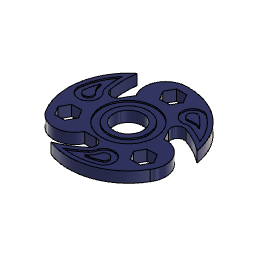
Fidget Spinner (Autodesk Fusion 360 design; units mm, degrees)
Autodesk Fusion 360 part; units mm, degrees
sketch "Sketch1" plane through (0, 0, 0) normal (0, 0, 1) x (1, 0, 0)
  circle A0 centre (0, 0) radius 4
  circle A1 centre (0, 0) radius 11
  circle A2 centre (0, 0) radius 13.5
  circle A3 centre (0, 0) radius 17.5
  line L0 (-18.6674, 12.667) -> (-14.3305, 20.1788)
  line L1 (20.3037, 9.833) -> (24.5374, 2.5)
  line L2 (-10.1036, -22.5) -> (-1.6363, -22.5)
  arc A4 (38.9711, 22.5) -> (0, 45) centre (0, 0) ccw
  arc A5 (44.4373, 7.0943) -> (38.9711, 22.5) centre (0, 0) ccw
  arc A6 (0, 45) -> (-14.3305, 20.1788) centre (-0.9803, 29.0185) ccw
  arc A7 (44.4373, 7.0943) -> (26.3003, 17.0471) centre (4.9389, -43.3819) ccw
  line L3 (-3.4682, 39.5482) -> (-7.0418, 32.948)
  line L4 (-7.0418, 32.948) -> (-3.1126, 26.5531)
  line L5 (-3.1126, 26.5531) -> (4.3902, 26.7584)
  line L6 (4.3902, 26.7584) -> (7.9637, 33.3586)
  line L7 (7.9637, 33.3586) -> (4.0345, 39.7535)
  line L8 (4.0345, 39.7535) -> (-3.4682, 39.5482)
  arc A8 (26.3003, 17.0471) -> (20.3037, 9.833) centre (24.6338, 12.333) ccw
  arc A9 (-38.9711, -22.5) -> (-10.3101, -22.5) centre (-24.6406, -15.3583) ccw
  arc A10 (-38.9711, 22.5) -> (-38.9711, -22.5) centre (0, 0) ccw
  line L9 (-32.8713, -9.7825) -> (-36.4448, -16.3828)
  line L10 (-36.4448, -16.3828) -> (-32.5156, -22.7777)
  line L11 (-32.5156, -22.7777) -> (-25.0129, -22.5723)
  line L12 (-25.0129, -22.5723) -> (-21.4394, -15.9721)
  line L13 (-21.4394, -15.9721) -> (-25.3686, -9.5772)
  line L14 (-25.3686, -9.5772) -> (-32.8713, -9.7825)
  arc A11 (-28.3625, 34.9366) -> (-38.9711, 22.5) centre (0, 0) ccw
  arc A12 (-28.3625, 34.9366) -> (-27.9133, 14.2531) centre (35.1004, 25.9682) ccw
  arc A13 (-27.9133, 14.2531) -> (-18.6674, 12.667) centre (-22.9976, 15.167) ccw
  line L15 (-18.6674, 12.667) -> (-14.4338, 20)
  line L16 (24.5374, 2.5) -> (20.3037, 9.833)
  line L17 (-1.6363, -22.5) -> (-10.3101, -22.5)
  arc A14 (38.9711, -22.5) -> (24.6406, 2.3212) centre (25.6209, -13.6603) ccw
  arc A15 (0, -45) -> (38.9711, -22.5) centre (0, 0) ccw
  line L18 (24.9076, -23.5761) -> (32.4103, -23.3708)
  line L19 (32.4103, -23.3708) -> (35.9839, -16.7705)
  line L20 (35.9839, -16.7705) -> (32.0547, -10.3756)
  line L21 (32.0547, -10.3756) -> (24.5519, -10.581)
  line L22 (24.5519, -10.581) -> (20.9784, -17.1812)
  line L23 (20.9784, -17.1812) -> (24.9076, -23.5761)
  arc A16 (-16.0748, -42.031) -> (0, -45) centre (0, 0) ccw
  arc A17 (-16.0748, -42.031) -> (1.6131, -31.3002) centre (-40.0393, 17.4137) ccw
  arc A18 (1.6131, -31.3002) -> (-1.6363, -22.5) centre (-1.6363, -27.5) ccw
  line L24 (-1.6363, -22.5) -> (-10.1036, -22.5)
  line L25 (-14.4338, 20) -> (-18.6674, 12.667)
  line L26 (20.3037, 9.833) -> (24.6406, 2.3212)
  dimension "d2" = 8
  dimension "d4" = 22
  dimension "d5" = 2.5
  dimension "d6" = 35
  dimension "d12" = 22
  dimension "d13" = 8
  dimension "d14" = 5
  constraint coincident A0.centre A1.centre
  constraint coincident A6.start A4
  constraint tangent L1 A8
  constraint tangent A7 A8
  measures "d2" diameter of A0
  measures "d4" diameter of A1
  measures "d6" diameter of A3
  measures "d12" diameter of A1
  measures "d13" diameter of A0
  measures "d14" radius of A8
sketch "Sketch2" plane through (0, 0, 0) normal (0, 0, 1) x (1, 0, 0)
extrude "Extrude1" add sketch "Sketch1" along normal blind 8 contours A2 | A3 | L0 L1 L2 A4 A5 A6 A7 A8 A9 A10 A11 A12 A13 L15 L16 L17 A14 A15 A16 A17 A18 L24 L25 L26
sketch "Sketch3" plane through (0, 0, 8) normal (0, 0, 1) x (-1, 0, 0)
  line L0 (32.8713, 9.7825) -> (25.3686, 9.5772)
  line L1 (25.3686, 9.5772) -> (21.4394, 15.9721)
  line L2 (21.4394, 15.9721) -> (25.0129, 22.5723)
  line L3 (25.0129, 22.5723) -> (32.5156, 22.7777)
  line L4 (32.5156, 22.7777) -> (36.4448, 16.3828)
  line L5 (36.4448, 16.3828) -> (32.8713, 9.7825)
  line L6 (3.4682, -39.5482) -> (-4.0345, -39.7535)
  line L7 (-4.0345, -39.7535) -> (-7.9637, -33.3586)
  line L8 (-7.9637, -33.3586) -> (-4.3902, -26.7584)
  line L9 (-4.3902, -26.7584) -> (3.1126, -26.5531)
  line L10 (3.1126, -26.5531) -> (7.0418, -32.948)
  line L11 (7.0418, -32.948) -> (3.4682, -39.5482)
  circle A0 centre (0, 0) radius 11
  line L12 (-24.9076, 23.5761) -> (-20.9784, 17.1812)
  line L13 (-20.9784, 17.1812) -> (-24.5519, 10.581)
  line L14 (-24.5519, 10.581) -> (-32.0547, 10.3756)
  line L15 (-32.0547, 10.3756) -> (-35.9839, 16.7705)
  line L16 (-35.9839, 16.7705) -> (-32.4103, 23.3708)
  line L17 (-32.4103, 23.3708) -> (-24.9076, 23.5761)
  arc A1 (-44.4373, -7.0943) -> (0, -45) centre (0, 0) ccw
  arc A2 (0, -45) -> (14.3305, -20.1788) centre (0.9803, -29.0185) ccw
  line L18 (14.3305, -20.1788) -> (18.6674, -12.667)
  arc A3 (27.9133, -14.2531) -> (18.6674, -12.667) centre (22.9976, -15.167) ccw
  arc A4 (28.3625, -34.9366) -> (27.9133, -14.2531) centre (-35.1004, -25.9682) ccw
  arc A5 (28.3625, -34.9366) -> (38.9711, 22.5) centre (0, 0) ccw
  arc A6 (38.9711, 22.5) -> (10.3101, 22.5) centre (24.6406, 15.3583) ccw
  line L19 (10.3101, 22.5) -> (1.6363, 22.5)
  arc A7 (-1.6131, 31.3002) -> (1.6363, 22.5) centre (1.6363, 27.5) ccw
  arc A8 (16.0748, 42.031) -> (-1.6131, 31.3002) centre (40.0393, -17.4137) ccw
  arc A9 (16.0748, 42.031) -> (-38.9711, 22.5) centre (0, 0) ccw
  arc A10 (-38.9711, 22.5) -> (-24.6406, -2.3212) centre (-25.6209, 13.6603) ccw
  line L20 (-24.6406, -2.3212) -> (-20.3037, -9.833)
  arc A11 (-26.3003, -17.0471) -> (-20.3037, -9.833) centre (-24.6338, -12.333) ccw
  arc A12 (-44.4373, -7.0943) -> (-26.3003, -17.0471) centre (-4.9389, 43.3819) ccw
  arc A13 (30.8628, -13.7048) -> (28.0927, -8.9994) centre (22.9976, -15.167) ccw
  arc A14 (31.9813, -27.2249) -> (30.8628, -13.7048) centre (-35.1004, -25.9682) ccw
  arc A15 (31.9813, -27.2249) -> (41.8312, -3.7617) centre (0, 0) ccw
  arc A16 (7.5868, 41.3091) -> (-3.5627, 33.5804) centre (40.0393, -17.4137) ccw
  arc A17 (41.8312, -3.7617) -> (29.2995, -10.239) centre (34.1663, -4.2937) ccw
  arc A18 (31.9813, -27.2249) -> (41.8312, -3.7617) centre (0, 0) ccw
  arc A19 (7.5868, 41.3091) -> (-17.6578, 38.1078) centre (0, 0) ccw
  arc A20 (7.5868, 41.3091) -> (-3.5627, 33.5804) centre (40.0393, -17.4137) ccw
  arc A21 (-17.6578, 38.1078) -> (-5.7825, 30.4936) centre (-13.3647, 31.7358) ccw
  arc A22 (-3.5627, 33.5804) -> (-6.2526, 28.8287) centre (1.6363, 27.5) ccw
  arc A23 (-39.5681, -14.0842) -> (-24.1734, -34.346) centre (0, 0) ccw
  arc A24 (-39.5681, -14.0842) -> (-27.3001, -19.8756) centre (-4.9389, 43.3819) ccw
  arc A25 (-24.1734, -34.346) -> (-23.517, -20.2546) centre (-20.8016, -27.4421) ccw
  arc A26 (-27.3001, -19.8756) -> (-21.8401, -19.8293) centre (-24.6338, -12.333) ccw
  dimension "d22" = 360
  constraint coincident A13 A17.end
  constraint concentric A3 A13
  constraint concentric A4 A14
  constraint concentric A5 A15
  constraint concentric A8 A16
  constraint tangent A13 A14
  constraint coincident A17 A13.end
extrude "Extrude2" cut sketch "Sketch3" against normal blind 1 contours A13 A14 A15 A17 A18 | A16 A19 A20 A21 A22 | A23 A24 A25 A26
sketch "Sketch4" plane through (0, 0, 8) normal (0, 0, 1) x (-1, 0, 0)
  arc A0 (31.9813, -27.2249) -> (41.8312, -3.7617) centre (0, 0) ccw
  arc A1 (31.9813, -27.2249) -> (30.8628, -13.7048) centre (-35.1004, -25.9682) ccw
  arc A2 (30.8628, -13.7048) -> (28.0927, -8.9994) centre (22.9976, -15.167) ccw
  arc A3 (41.8312, -3.7617) -> (28.0927, -8.9994) centre (34.1663, -4.2937) ccw
  arc A4 (-24.1734, -34.346) -> (-21.8401, -19.8293) centre (-20.8016, -27.4421) ccw
  arc A5 (-39.5681, -14.0842) -> (-24.1734, -34.346) centre (0, 0) ccw
  arc A6 (-39.5681, -14.0842) -> (-27.3001, -19.8756) centre (-4.9389, 43.3819) ccw
  arc A7 (-27.3001, -19.8756) -> (-21.8401, -19.8293) centre (-24.6338, -12.333) ccw
  arc A8 (-17.6578, 38.1078) -> (-6.2526, 28.8287) centre (-13.3647, 31.7358) ccw
  arc A9 (7.5868, 41.3091) -> (-17.6578, 38.1078) centre (0, 0) ccw
  arc A10 (7.5868, 41.3091) -> (-3.5627, 33.5804) centre (40.0393, -17.4137) ccw
  arc A11 (-3.5627, 33.5804) -> (-6.2526, 28.8287) centre (1.6363, 27.5) ccw
  line L0 (32.8713, 9.7825) -> (25.3686, 9.5772)
  line L1 (25.3686, 9.5772) -> (21.4394, 15.9721)
  line L2 (21.4394, 15.9721) -> (25.0129, 22.5723)
  line L3 (25.0129, 22.5723) -> (32.5156, 22.7777)
  line L4 (32.5156, 22.7777) -> (36.4448, 16.3828)
  line L5 (36.4448, 16.3828) -> (32.8713, 9.7825)
  line L6 (3.4682, -39.5482) -> (-4.0345, -39.7535)
  line L7 (-4.0345, -39.7535) -> (-7.9637, -33.3586)
  line L8 (-7.9637, -33.3586) -> (-4.3902, -26.7584)
  line L9 (-4.3902, -26.7584) -> (3.1126, -26.5531)
  line L10 (3.1126, -26.5531) -> (7.0418, -32.948)
  line L11 (7.0418, -32.948) -> (3.4682, -39.5482)
  circle A12 centre (0, 0) radius 11
  line L12 (-24.9076, 23.5761) -> (-20.9784, 17.1812)
  line L13 (-20.9784, 17.1812) -> (-24.5519, 10.581)
  line L14 (-24.5519, 10.581) -> (-32.0547, 10.3756)
  line L15 (-32.0547, 10.3756) -> (-35.9839, 16.7705)
  line L16 (-35.9839, 16.7705) -> (-32.4103, 23.3708)
  line L17 (-32.4103, 23.3708) -> (-24.9076, 23.5761)
  arc A13 (-44.4373, -7.0943) -> (0, -45) centre (0, 0) ccw
  arc A14 (0, -45) -> (14.3305, -20.1788) centre (0.9803, -29.0185) ccw
  line L18 (14.3305, -20.1788) -> (18.6674, -12.667)
  arc A15 (27.9133, -14.2531) -> (18.6674, -12.667) centre (22.9976, -15.167) ccw
  arc A16 (28.3625, -34.9366) -> (27.9133, -14.2531) centre (-35.1004, -25.9682) ccw
  arc A17 (28.3625, -34.9366) -> (38.9711, 22.5) centre (0, 0) ccw
  arc A18 (38.9711, 22.5) -> (10.3101, 22.5) centre (24.6406, 15.3583) ccw
  line L19 (10.3101, 22.5) -> (1.6363, 22.5)
  arc A19 (-1.6131, 31.3002) -> (1.6363, 22.5) centre (1.6363, 27.5) ccw
  arc A20 (16.0748, 42.031) -> (-1.6131, 31.3002) centre (40.0393, -17.4137) ccw
  arc A21 (16.0748, 42.031) -> (-38.9711, 22.5) centre (0, 0) ccw
  arc A22 (-38.9711, 22.5) -> (-24.6406, -2.3212) centre (-25.6209, 13.6603) ccw
  line L20 (-24.6406, -2.3212) -> (-20.3037, -9.833)
  arc A23 (-26.3003, -17.0471) -> (-20.3037, -9.833) centre (-24.6338, -12.333) ccw
  arc A24 (-44.4373, -7.0943) -> (-26.3003, -17.0471) centre (-4.9389, 43.3819) ccw
  circle A25 centre (0, 0) radius 15
  circle A26 centre (0, 0) radius 20
  constraint coincident A0.centre A5.centre
  constraint concentric A25 A26
sketch "Sketch5" plane through (0, 0, 8) normal (0, 0, 1) x (-1, 0, 0)
extrude "Extrude3" cut sketch "Sketch4" against normal blind 1 contours A26
sketch "Sketch6" plane through (0, 0, 0) normal (0, 0, -1) x (1, 0, 0)
  line L0 (-25.3686, 9.5772) -> (-32.8713, 9.7825)
  line L1 (-32.8713, 9.7825) -> (-36.4448, 16.3828)
  line L2 (-36.4448, 16.3828) -> (-32.5156, 22.7777)
  line L3 (-32.5156, 22.7777) -> (-25.0129, 22.5723)
  line L4 (-25.0129, 22.5723) -> (-21.4394, 15.9721)
  line L5 (-21.4394, 15.9721) -> (-25.3686, 9.5772)
  line L6 (4.0345, -39.7535) -> (-3.4682, -39.5482)
  line L7 (-3.4682, -39.5482) -> (-7.0418, -32.948)
  line L8 (-7.0418, -32.948) -> (-3.1126, -26.5531)
  line L9 (-3.1126, -26.5531) -> (4.3902, -26.7584)
  line L10 (4.3902, -26.7584) -> (7.9637, -33.3586)
  line L11 (7.9637, -33.3586) -> (4.0345, -39.7535)
  circle A0 centre (0, 0) radius 11
  line L12 (20.9784, 17.1812) -> (24.9076, 23.5761)
  line L13 (24.9076, 23.5761) -> (32.4103, 23.3708)
  line L14 (32.4103, 23.3708) -> (35.9839, 16.7705)
  line L15 (35.9839, 16.7705) -> (32.0547, 10.3756)
  line L16 (32.0547, 10.3756) -> (24.5519, 10.581)
  line L17 (24.5519, 10.581) -> (20.9784, 17.1812)
  arc A1 (0, -45) -> (44.4373, -7.0943) centre (0, 0) ccw
  arc A2 (26.3003, -17.0471) -> (44.4373, -7.0943) centre (4.9389, 43.3819) ccw
  arc A3 (20.3037, -9.833) -> (26.3003, -17.0471) centre (24.6338, -12.333) ccw
  line L18 (20.3037, -9.833) -> (24.6406, -2.3212)
  arc A4 (24.6406, -2.3212) -> (38.9711, 22.5) centre (25.6209, 13.6603) ccw
  arc A5 (38.9711, 22.5) -> (-16.0748, 42.031) centre (0, 0) ccw
  arc A6 (1.6131, 31.3002) -> (-16.0748, 42.031) centre (-40.0393, -17.4137) ccw
  arc A7 (-1.6363, 22.5) -> (1.6131, 31.3002) centre (-1.6363, 27.5) ccw
  line L19 (-1.6363, 22.5) -> (-10.3101, 22.5)
  arc A8 (-10.3101, 22.5) -> (-38.9711, 22.5) centre (-24.6406, 15.3583) ccw
  arc A9 (-38.9711, 22.5) -> (-28.3625, -34.9366) centre (0, 0) ccw
  arc A10 (-27.9133, -14.2531) -> (-28.3625, -34.9366) centre (35.1004, -25.9682) ccw
  arc A11 (-18.6674, -12.667) -> (-27.9133, -14.2531) centre (-22.9976, -15.167) ccw
  line L20 (-18.6674, -12.667) -> (-14.3305, -20.1788)
  arc A12 (-14.3305, -20.1788) -> (0, -45) centre (-0.9803, -29.0185) ccw
  arc A13 (-28.2531, -9.1355) -> (-30.8628, -13.7048) centre (-22.9976, -15.167) ccw
  arc A14 (-30.8628, -13.7048) -> (-31.9813, -27.2249) centre (35.1004, -25.9682) ccw
  arc A15 (-41.8312, -3.7617) -> (-31.9813, -27.2249) centre (0, 0) ccw
  arc A16 (-29.2995, -10.239) -> (-41.8312, -3.7617) centre (-34.2643, -4.4832) ccw
  arc A17 (22.0381, -19.9001) -> (27.3001, -19.8756) centre (24.6338, -12.333) ccw
  arc A18 (27.3001, -19.8756) -> (39.5681, -14.0842) centre (4.9389, 43.3819) ccw
  arc A19 (24.1734, -34.346) -> (39.5681, -14.0842) centre (0, 0) ccw
  arc A20 (23.517, -20.2546) -> (24.1734, -34.346) centre (21.0147, -27.4321) ccw
  arc A21 (6.215, 29.0357) -> (3.5627, 33.5804) centre (-1.6363, 27.5) ccw
  arc A22 (3.5627, 33.5804) -> (-7.5868, 41.3091) centre (-40.0393, -17.4137) ccw
  arc A23 (17.6578, 38.1078) -> (-7.5868, 41.3091) centre (0, 0) ccw
  arc A24 (5.7825, 30.4936) -> (17.6578, 38.1078) centre (13.2496, 31.9154) ccw
  dimension "d29" = 360
  constraint coincident A13 A16.start
  constraint concentric A11 A13
  constraint concentric A10 A14
  constraint concentric A9 A15
  constraint tangent A13 A14
  constraint coincident A16 A13.start
extrude "Extrude4" cut sketch "Sketch6" against normal blind 1 contours A13 A14 A15 A16 | A17 A18 A19 A20 | A21 A22 A23 A24
sketch "Sketch7" plane through (0, 0, 0) normal (0, 0, -1) x (1, 0, 0)
  arc A0 (3.5627, 33.5804) -> (-7.5868, 41.3091) centre (-40.0393, -17.4137) ccw
  arc A1 (17.6578, 38.1078) -> (-7.5868, 41.3091) centre (0, 0) ccw
  arc A2 (6.215, 29.0357) -> (17.6578, 38.1078) centre (13.2496, 31.9154) ccw
  arc A3 (6.215, 29.0357) -> (3.5627, 33.5804) centre (-1.6363, 27.5) ccw
  arc A4 (27.3001, -19.8756) -> (39.5681, -14.0842) centre (4.9389, 43.3819) ccw
  arc A5 (24.1734, -34.346) -> (39.5681, -14.0842) centre (0, 0) ccw
  arc A6 (22.0381, -19.9001) -> (24.1734, -34.346) centre (21.0147, -27.4321) ccw
  arc A7 (22.0381, -19.9001) -> (27.3001, -19.8756) centre (24.6338, -12.333) ccw
  arc A8 (-30.8628, -13.7048) -> (-31.9813, -27.2249) centre (35.1004, -25.9682) ccw
  arc A9 (-41.8312, -3.7617) -> (-31.9813, -27.2249) centre (0, 0) ccw
  arc A10 (-28.2531, -9.1355) -> (-41.8312, -3.7617) centre (-34.2643, -4.4832) ccw
  arc A11 (-28.2531, -9.1355) -> (-30.8628, -13.7048) centre (-22.9976, -15.167) ccw
  line L0 (-25.3686, 9.5772) -> (-32.8713, 9.7825)
  line L1 (-32.8713, 9.7825) -> (-36.4448, 16.3828)
  line L2 (-36.4448, 16.3828) -> (-32.5156, 22.7777)
  line L3 (-32.5156, 22.7777) -> (-25.0129, 22.5723)
  line L4 (-25.0129, 22.5723) -> (-21.4394, 15.9721)
  line L5 (-21.4394, 15.9721) -> (-25.3686, 9.5772)
  line L6 (4.0345, -39.7535) -> (-3.4682, -39.5482)
  line L7 (-3.4682, -39.5482) -> (-7.0418, -32.948)
  line L8 (-7.0418, -32.948) -> (-3.1126, -26.5531)
  line L9 (-3.1126, -26.5531) -> (4.3902, -26.7584)
  line L10 (4.3902, -26.7584) -> (7.9637, -33.3586)
  line L11 (7.9637, -33.3586) -> (4.0345, -39.7535)
  circle A12 centre (0, 0) radius 11
  line L12 (20.9784, 17.1812) -> (24.9076, 23.5761)
  line L13 (24.9076, 23.5761) -> (32.4103, 23.3708)
  line L14 (32.4103, 23.3708) -> (35.9839, 16.7705)
  line L15 (35.9839, 16.7705) -> (32.0547, 10.3756)
  line L16 (32.0547, 10.3756) -> (24.5519, 10.581)
  line L17 (24.5519, 10.581) -> (20.9784, 17.1812)
  arc A13 (0, -45) -> (44.4373, -7.0943) centre (0, 0) ccw
  arc A14 (26.3003, -17.0471) -> (44.4373, -7.0943) centre (4.9389, 43.3819) ccw
  arc A15 (20.3037, -9.833) -> (26.3003, -17.0471) centre (24.6338, -12.333) ccw
  line L18 (20.3037, -9.833) -> (24.6406, -2.3212)
  arc A16 (24.6406, -2.3212) -> (38.9711, 22.5) centre (25.6209, 13.6603) ccw
  arc A17 (38.9711, 22.5) -> (-16.0748, 42.031) centre (0, 0) ccw
  arc A18 (1.6131, 31.3002) -> (-16.0748, 42.031) centre (-40.0393, -17.4137) ccw
  arc A19 (-1.6363, 22.5) -> (1.6131, 31.3002) centre (-1.6363, 27.5) ccw
  line L19 (-1.6363, 22.5) -> (-10.3101, 22.5)
  arc A20 (-10.3101, 22.5) -> (-38.9711, 22.5) centre (-24.6406, 15.3583) ccw
  arc A21 (-38.9711, 22.5) -> (-28.3625, -34.9366) centre (0, 0) ccw
  arc A22 (-27.9133, -14.2531) -> (-28.3625, -34.9366) centre (35.1004, -25.9682) ccw
  arc A23 (-18.6674, -12.667) -> (-27.9133, -14.2531) centre (-22.9976, -15.167) ccw
  line L20 (-18.6674, -12.667) -> (-14.3305, -20.1788)
  arc A24 (-14.3305, -20.1788) -> (0, -45) centre (-0.9803, -29.0185) ccw
  circle A25 centre (0, 0) radius 13.8811
  circle A26 centre (0, 0) radius 20
  constraint concentric A1 A25
  constraint concentric A1 A26
extrude "Extrude5" cut sketch "Sketch7" against normal blind 1 contours A26
sketch "Sketch8" plane through (0, 0, 7) normal (0, 0, 1) x (-1, 0, 0)
  arc A0 (31.9813, -27.2249) -> (30.8628, -13.7048) centre (-35.1004, -25.9682) ccw
  arc A1 (31.9813, -27.2249) -> (41.8312, -3.7617) centre (0, 0) ccw
  arc A2 (41.8312, -3.7617) -> (28.0927, -8.9994) centre (34.1663, -4.2937) ccw
  arc A3 (30.8628, -13.7048) -> (28.0927, -8.9994) centre (22.9976, -15.167) ccw
  arc A4 (37.8124, -3.7713) -> (31.0693, -6.2875) centre (34.1663, -4.2937) ccw
  arc A5 (34.7954, -12.9737) -> (31.0693, -6.2875) centre (22.9976, -15.167) ccw
  arc A6 (35.0797, -14.6087) -> (34.7954, -12.9737) centre (-35.1004, -25.9682) ccw
  arc A7 (35.0797, -14.6087) -> (37.8124, -3.7713) centre (0, 0) ccw
  arc A8 (-4.8883, 37.6843) -> (-15.6402, 34.6321) centre (0, 0) ccw
  arc A9 (-4.8883, 37.6843) -> (-6.1622, 36.6206) centre (40.0393, -17.4137) ccw
  arc A10 (-6.1622, 36.6206) -> (-10.0895, 30.0506) centre (1.6363, 27.5) ccw
  arc A11 (-15.6402, 34.6321) -> (-10.0895, 30.0506) centre (-13.3647, 31.7358) ccw
  arc A12 (-30.1914, -23.0755) -> (-22.1722, -30.8609) centre (0, 0) ccw
  arc A13 (-30.1914, -23.0755) -> (-28.6332, -23.6469) centre (-4.9389, 43.3819) ccw
  arc A14 (-28.6332, -23.6469) -> (-20.9798, -23.7631) centre (-24.6338, -12.333) ccw
  arc A15 (-22.1722, -30.8609) -> (-20.9798, -23.7631) centre (-20.8016, -27.4421) ccw
  dimension "d34" = 4
  dimension "d36" = 360
sketch "Sketch9" plane through (0, 0, 7) normal (0, 0, 1) x (-1, 0, 0)
extrude "Extrude6" add sketch "Sketch8" along normal blind 1 contours A4 A5 A6 A7 | A8 A9 A10 A11 | A12 A13 A14 A15
sketch "Sketch10" plane through (0, 0, 1) normal (0, 0, -1) x (1, 0, 0)
  arc A0 (24.1734, -34.346) -> (39.5681, -14.0842) centre (0, 0) ccw
  arc A1 (27.3001, -19.8756) -> (39.5681, -14.0842) centre (4.9389, 43.3819) ccw
  arc A2 (22.0381, -19.9001) -> (27.3001, -19.8756) centre (24.6338, -12.333) ccw
  arc A3 (22.0381, -19.9001) -> (24.1734, -34.346) centre (21.0147, -27.4321) ccw
  arc A4 (28.6332, -23.6469) -> (30.1914, -23.0755) centre (4.9389, 43.3819) ccw
  arc A5 (22.2222, -30.8249) -> (30.1914, -23.0755) centre (0, 0) ccw
  arc A6 (21.2186, -23.8367) -> (22.2222, -30.8249) centre (21.0147, -27.4321) ccw
  arc A7 (21.2186, -23.8367) -> (28.6332, -23.6469) centre (24.6338, -12.333) ccw
  arc A8 (10.0339, 30.2942) -> (6.1622, 36.6206) centre (-1.6363, 27.5) ccw
  arc A9 (6.1622, 36.6206) -> (4.8883, 37.6843) centre (-40.0393, -17.4137) ccw
  arc A10 (15.5841, 34.6574) -> (4.8883, 37.6843) centre (0, 0) ccw
  arc A11 (10.0339, 30.2942) -> (15.5841, 34.6574) centre (13.2496, 31.9154) ccw
  arc A12 (-31.2525, -6.4575) -> (-34.7954, -12.9737) centre (-22.9976, -15.167) ccw
  arc A13 (-34.7954, -12.9737) -> (-35.0797, -14.6087) centre (35.1004, -25.9682) ccw
  arc A14 (-37.8062, -3.8325) -> (-35.0797, -14.6087) centre (0, 0) ccw
  arc A15 (-31.2525, -6.4575) -> (-37.8062, -3.8325) centre (-34.2643, -4.4832) ccw
  dimension "d39" = -4
  dimension "d41" = 360
extrude "Extrude7" add sketch "Sketch10" along normal blind 1 contours A4 A5 A6 A7 | A8 A9 A10 A11 | A12 A13 A14 A15
